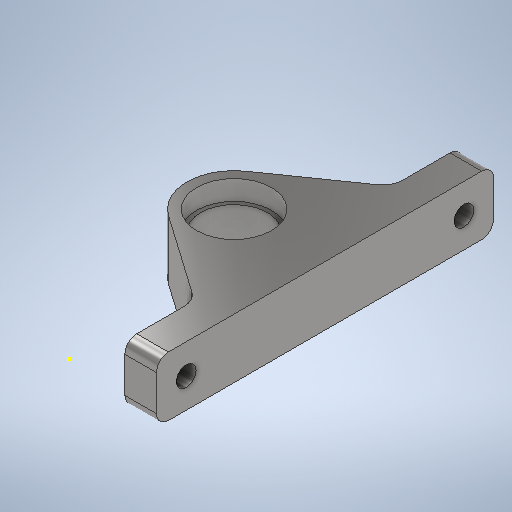
# Autodesk Inventor part: mancal[1]
Saved by Autodesk Inventor 2025 (Build 290162010, 162A)
## iProperties
Created: 2024-09-25
Part Number: mancal[1]
Material: Steel, Mild
Document SubType Name: Modeling
Designer: IFSP
Density: 7.85 g/cm^3
Appearance: Semi-Polished
Author: IFSP
Autodesk Inventor part; units mm, degrees
ref_plane "YZ Plane" through (0, 0, 0) normal (1, 0, 0) x (0, 1, 0)
ref_plane "XZ Plane" through (0, 0, 0) normal (0, 1, 0) x (-1, 0, 0)
ref_plane "XY Plane" through (0, 0, 0) normal (0, 0, 1) x (1, 0, 0)
sketch "Sketch1" plane through (0, 0, 0) normal (0, 1, 0) x (-1, 0, 0)
  circle A0 centre (0, 0) radius 9.45
  circle A1 centre (0, 0) radius 8.45
  line L0 (15.45, 25) -> (15.45, -25)
  line L1 (-20, 0) -> (-15, 0)
  line L2 (-15, 0) -> (-15, 25)
  line L3 (-15, 25) -> (-20, 25)
  line L4 (-20, 25) -> (-20, 0)
  line L5 (-20, 0) -> (-15, 0)
  line L6 (-15, 0) -> (-15, -25)
  line L7 (-15, -25) -> (-20, -25)
  line L8 (-20, -25) -> (-20, 0)
  line L9 (15.45, 25) -> (-20, 25)
  line L10 (-20, 25) -> (-20, -25)
  line L11 (-20, -25) -> (15.45, -25)
  line L12 (15.45, -25) -> (15.45, 25)
  point P0 (15.45, 0)
  dimension "d0" = 18.9
  dimension "d1" = 16.9
  dimension "d7" = 5
  dimension "d8" = 20
  constraints: 26 end point, 6 parallel, 3 horizontal, 3 perpendicular, 2 centre point, 2 coincident
  measures "d0" diameter of A0
  measures "d1" diameter of A1
  measures "d7" distance of L3.end L2.end
  measures "d8" distance from line of L8 point (0, 0)
extrude "Extrusion1" add sketch "Sketch1" along normal blind 10 contours L0 L11 L6 L2 L9 | L2 L1 L4 L3 | L7 L8 L1 L6
extrude "Extrusion2" add sketch "Sketch1" along normal blind 4.9 contours A0
sketch "Sketch2" plane through (0, 10, 0) normal (0, 1, 0) x (1, 0, 0)
  circle A0 centre (0, 0) radius 11.9
  line L0 (-15.45, -25) -> (20, -25) projected
  line L1 (20, 25) -> (-15.45, 25) projected
  line L2 (20, -25) -> (15, -25)
  line L3 (15, -25) -> (15, 25)
  line L4 (15, 25) -> (20, 25)
  line L5 (20, 25) -> (20, -25)
  line L6 (-15.45, 25) -> (-15.45, -25) projected
  line L7 (20, -25) -> (-15.45, -25)
  line L8 (-15.45, -25) -> (-15.45, 25)
  line L9 (-15.45, 25) -> (20, 25)
  line L10 (20, 25) -> (20, -25)
  point P0 (-6.8165, -9.7543)
  point P1 (-6.8165, 9.7543)
  dimension "d13" = 23.8
  dimension "d14" = 5
  constraints: 16 end point, 4 parallel, 2 horizontal, 2 perpendicular, 2 point on circle, 1 centre point, 1 coincident, 1 point on line
  measures "d13" diameter of A0
  measures "d14" distance of L3.end L4.end
sketch "Sketch7" plane through (20, 0, -25) normal (0, 0, -1) x (-1, 0, 0)
  line L0 (35.45, 0) -> (35.45, 10) projected
  line L1 (0, 0) -> (35.45, 0)
  line L2 (35.45, 0) -> (35.45, 10)
  line L3 (35.45, 10) -> (0, 10)
  line L4 (0, 10) -> (0, 0)
  point P0 (20, 0)
  constraints: 8 end point, 2 parallel, 1 horizontal, 1 perpendicular
extrude "Extrusion7" add sketch "Sketch7" along normal blind 10
sketch "Sketch8" plane through (-15.45, 0, 25) normal (0, 0, 1) x (1, 0, 0)
  line L0 (35.45, 0) -> (35.45, 10) projected
  line L1 (0, 0) -> (0, 10) projected
  line L2 (35.45, 0) -> (0, 0)
  line L3 (0, 0) -> (0, 10)
  line L4 (0, 10) -> (35.45, 10)
  line L5 (35.45, 10) -> (35.45, 0)
  point P0 (15.45, 0)
  constraints: 8 end point, 2 parallel, 1 horizontal, 1 perpendicular
extrude "Extrusion8" add sketch "Sketch8" along normal blind 10
sketch "Sketch9" plane through (0, 10, 0) normal (0, 1, 0) x (1, 0, 0)
  circle A0 centre (0, 0) radius 11.9 projected
  line L0 (15, -25) -> (15, 25) projected
  line L1 (15, -25) -> (-6.8165, -9.7543)
  line L2 (15, 25) -> (-6.8165, 9.7543)
  line L3 (20, 35) -> (20, -35) projected
  line L4 (20, 25) -> (15, 25)
  line L5 (15, 25) -> (15, 35)
  line L6 (15, 35) -> (20, 35)
  line L7 (20, 35) -> (20, 25)
  line L8 (20, -25) -> (15, -25)
  line L9 (15, -25) -> (15, -35)
  line L10 (15, -35) -> (20, -35)
  line L11 (20, -35) -> (20, -25)
  line L12 (15, -25) -> (15, 25)
  line L13 (-15.45, -35) -> (-15.45, 35) projected
  line L14 (-15.45, 25) -> (15, 25)
  line L15 (15, -25) -> (-15.45, -25)
  line L16 (-15.45, -25) -> (-15.45, 25)
  line L17 (15, -25) -> (-15.45, -25)
  line L18 (-15.45, -25) -> (-15.45, -35)
  line L19 (-15.45, -35) -> (15, -35)
  line L20 (15, -35) -> (15, -25)
  line L21 (20, 35) -> (-15.45, 35) projected
  line L22 (15, 25) -> (-15.45, 25)
  line L23 (-15.45, 25) -> (-15.45, 35)
  line L24 (-15.45, 35) -> (15, 35)
  line L25 (15, 35) -> (15, 25)
  point P0 (15, 25)
  dimension "d27" = 10
  constraints: 44 end point, 9 parallel, 5 perpendicular, 4 horizontal, 4 point on line, 2 collinear, 2 point on circle, 2 tangent
  measures "d27" distance of L4.end L5.end
extrude "Extrusion9" cut sketch "Sketch9" against normal blind 10 contours A0 L1 L15 L13 L14 L2
extrude "Extrusion10" cut sketch "Sketch9" against normal blind 10 contours L14 L13 L21 L5 | L9 L19 L13 L15
fillet "Fillet1" radius 5 2 edges at (15, 5, 25) (15, 5, -25)
sketch "Sketch10" plane through (-15.45, 0, 35) normal (0, 0, 1) x (1, 0, 0)
  line L0 (35.45, 10) -> (35.45, 0) projected
  line L1 (30.45, 10) -> (30.45, 0) projected
  line L2 (35.45, 0) -> (30.45, 0)
  line L3 (30.45, 0) -> (30.45, 10)
  line L4 (30.45, 10) -> (35.45, 10)
  line L5 (35.45, 10) -> (35.45, 0)
  point P0 (15.45, 0)
  constraints: 8 end point, 2 parallel, 1 horizontal, 1 perpendicular
extrude "Extrusion11" add sketch "Sketch10" along normal blind 2.606
sketch "Sketch11" plane through (20, 0, -35) normal (0, 0, -1) x (-1, 0, 0)
  line L0 (5, 10) -> (0, 10) projected
  line L1 (5, 10) -> (5, 0) projected
  line L2 (0, 10) -> (5, 10)
  line L3 (5, 10) -> (5, 0)
  line L4 (5, 0) -> (0, 0)
  line L5 (0, 0) -> (0, 10)
  point P0 (20, 0)
  constraints: 8 end point, 2 parallel, 1 horizontal, 1 perpendicular
extrude "Extrusion12" add sketch "Sketch11" along normal blind 2.606
sketch "Sketch14" plane through (0, 10, 0) normal (0, 1, 0) x (1, 0, 0)
  circle A0 centre (0, 0) radius 9.45 projected
  line L0 (15, 37.606) -> (15, 27.6058) projected
  arc A1 (12.8641, 23.5074) -> (15, 27.6058) centre (10, 27.6058) ccw projected
  line L1 (12.8641, 23.5074) -> (-6.8165, 9.7543) projected
  arc A2 (-6.8165, 9.7543) -> (-6.8165, -9.7543) centre (0, 0) ccw projected
  line L2 (-6.8165, -9.7543) -> (12.8641, -23.5074) projected
  arc A3 (15, -27.6058) -> (12.8641, -23.5074) centre (10, -27.6058) ccw projected
  line L3 (15, -27.6058) -> (15, -37.606) projected
  line L4 (20, -37.606) -> (15, -37.606) projected
  line L5 (20, 37.606) -> (20, -37.606) projected
  line L6 (15, 37.606) -> (20, 37.606) projected
extrude "Extrusion15" add sketch "Sketch14" along normal blind 2
sketch "Sketch15" plane through (0, 0, 0) normal (0, -1, 0) x (1, 0, 0)
  line L0 (15, -27.6058) -> (15, -37.606) projected
  line L1 (20, -37.606) -> (15, -37.606) projected
  line L2 (20, 37.606) -> (20, -37.606) projected
  line L3 (15, 37.606) -> (20, 37.606) projected
  line L4 (15, 37.606) -> (15, 27.6058) projected
  arc A0 (12.8641, 23.5074) -> (15, 27.6058) centre (10, 27.6058) ccw projected
  line L5 (12.8641, 23.5074) -> (-6.8165, 9.7543) projected
  arc A1 (-6.8165, 9.7543) -> (-6.8165, -9.7543) centre (0, 0) ccw projected
  line L6 (-6.8165, -9.7543) -> (12.8641, -23.5074) projected
  arc A2 (15, -27.6058) -> (12.8641, -23.5074) centre (10, -27.6058) ccw projected
  circle A3 centre (0, 0) radius 8.45 projected
extrude "Extrusion16" add sketch "Sketch15" along normal blind 2
sketch "Sketch16" plane through (0, 4.9, 0) normal (0, 1, 0) x (1, 0, 0)
  circle A0 centre (0, 0) radius 9.45 projected
  circle A1 centre (0, 0) radius 8.45 projected
extrude "Extrusion17" add sketch "Sketch16" along normal blind 2.1
sketch "Sketch17" plane through (-15.45, 0, 37.606) normal (0, 0, 1) x (1, 0, 0)
  line L0 (35.45, 12) -> (35.45, -2) projected
  line L1 (30.45, 12) -> (35.45, 12) projected
  line L2 (30.45, -2) -> (30.45, 12) projected
  line L3 (35.45, -2) -> (30.45, -2) projected
  point P0 (15.45, 0)
extrude "Extrusion18" add sketch "Sketch17" along normal blind 4
sketch "Sketch18" plane through (20, 0, -37.606) normal (0, 0, -1) x (-1, 0, 0)
  line L0 (5, 12) -> (5, -2) projected
  line L1 (0, 12) -> (5, 12) projected
  line L2 (0, -2) -> (0, 12) projected
  line L3 (5, -2) -> (0, -2) projected
  point P0 (20, 0)
extrude "Extrusion19" add sketch "Sketch18" along normal blind 4
sketch "Sketch22" plane through (0, -2, 0) normal (0, -1, 0) x (1, 0, 0)
  arc A0 (-6.8165, 9.7543) -> (-6.8165, -9.7543) centre (0, 0) ccw projected
  line L0 (-6.8165, -9.7543) -> (12.8641, -23.5074) projected
  arc A1 (15, -27.6058) -> (12.8641, -23.5074) centre (10, -27.6058) ccw projected
  line L1 (15, -27.6058) -> (15, -41.606) projected
  line L2 (20, -41.606) -> (15, -41.606) projected
  line L3 (20, 41.606) -> (20, -41.606) projected
  line L4 (15, 41.606) -> (20, 41.606) projected
  line L5 (15, 27.6058) -> (15, 41.606) projected
  arc A2 (12.8641, 23.5074) -> (15, 27.6058) centre (10, 27.6058) ccw projected
  line L6 (12.8641, 23.5074) -> (-6.8165, 9.7543) projected
  circle A3 centre (0, 0) radius 8.45 projected
extrude "Extrusion22" add sketch "Sketch22" along normal blind 1
sketch "Sketch23" plane through (-15.45, 0, 41.606) normal (0, 0, 1) x (1, 0, 0)
  line L0 (30.45, 12) -> (30.45, -3) projected
  line L1 (35.45, -3) -> (30.45, -3) projected
  line L2 (35.45, 12) -> (35.45, -3) projected
  line L3 (35.45, 12) -> (30.45, 12) projected
  line L4 (35.45, 12) -> (35.45, -3) projected
  line L5 (30.45, -3) -> (35.45, -3) projected
  line L6 (30.45, 12) -> (30.45, -3) projected
  line L7 (30.45, 12) -> (35.45, 12) projected
  point P0 (15.45, 0)
sketch "Sketch24" plane through (-15.45, 0, 41.606) normal (0, 0, 1) x (1, 0, 0)
  point P0 (15.45, 0)
extrude "Extrusion23" add sketch "Sketch23" along normal blind 1
sketch "Sketch25" plane through (20, 0, -41.606) normal (0, 0, -1) x (-1, 0, 0)
  line L0 (0, 12) -> (0, -3) projected
  line L1 (5, -3) -> (0, -3) projected
  line L2 (5, 12) -> (5, -3) projected
  line L3 (5, 12) -> (0, 12) projected
  point P0 (20, 0)
extrude "Extrusion24" add sketch "Sketch25" along normal blind 1
sketch "Sketch26" plane through (15, -3, 27.6058) normal (-1, 0, 0) x (0, 0, 1)
  line L0 (0, 0) -> (0, 15) projected
  line L1 (0, 0) -> (15.0002, 0) projected
  line L2 (15.0002, 15) -> (15.0002, 0) projected
  line L3 (0, 15) -> (15.0002, 15) projected
  circle A0 centre (7.5001, 7.5) radius 2.5
  point P0 (-27.6058, 3)
  dimension "d67" = 5
  constraints: 1 centre point
  measures "d67" diameter of A0
extrude "Extrusion25" cut sketch "Sketch26" against normal up to surface (5 mm away) contours A0
sketch "Sketch27" plane through (15, -3, -27.6058) normal (-1, 0, 0) x (0, 0, 1)
  line L0 (0, 15) -> (0, 0) projected
  line L1 (0, 15) -> (-15.0002, 15) projected
  line L2 (-15.0002, 0) -> (-15.0002, 15) projected
  line L3 (0, 0) -> (-15.0002, 0) projected
  circle A0 centre (-7.5001, 7.5) radius 2.5
  point P0 (27.6058, 3)
  dimension "d70" = 5
  constraints: 1 centre point
  measures "d70" diameter of A0
extrude "Extrusion26" cut sketch "Sketch27" against normal up to surface (5 mm away) contours A0
fillet "Fillet4" radius 3 4 edges at (17.5, 12, 42.606) (17.5, -3, 42.606) (17.5, -3, -42.606) (17.5, 12, -42.606)
sketch "Sketch28" plane through (20, 0, 42.606) normal (1, 0, 0) x (0, 0, -1)
  arc A0 (85.212, 9) -> (82.212, 12) centre (82.212, 9) ccw projected
  line L0 (82.212, 12) -> (3, 12) projected
  arc A1 (3, 12) -> (0, 9) centre (3, 9) ccw projected
  line L1 (0, 0) -> (0, 9) projected
  arc A2 (0, 0) -> (3, -3) centre (3, 0) ccw projected
  line L2 (3, -3) -> (82.212, -3) projected
  arc A3 (82.212, -3) -> (85.212, 0) centre (82.212, 0) ccw projected
  line L3 (85.212, 9) -> (85.212, 0) projected
  circle A4 centre (77.7119, 4.5) radius 2.5 projected
  circle A5 centre (7.5001, 4.5) radius 2.5 projected
  point P0 (42.606, 0)
extrude "Extrusion27" add sketch "Sketch28" along normal blind 3
sketch "Sketch29" plane through (0, 12, 0) normal (0, 1, 0) x (1, 0, 0)
  line L0 (15, 39.606) -> (23, 39.606) projected
  line L1 (15, 27.6058) -> (15, 39.606) projected
  arc A0 (12.8641, 23.5074) -> (15, 27.6058) centre (10, 27.6058) ccw projected
  line L2 (12.8641, 23.5074) -> (-6.8165, 9.7543) projected
  arc A1 (-6.8165, 9.7543) -> (-6.8165, -9.7543) centre (0, 0) ccw projected
  line L3 (-6.8165, -9.7543) -> (12.8641, -23.5074) projected
  arc A2 (15, -27.6058) -> (12.8641, -23.5074) centre (10, -27.6058) ccw projected
  line L4 (15, -27.6058) -> (15, -39.606) projected
  line L5 (23, -39.606) -> (15, -39.606) projected
  line L6 (23, 39.606) -> (23, -39.606) projected
  circle A3 centre (0, 0) radius 9.45 projected
  circle A4 centre (0, 0) radius 8.45 projected
  line L7 (15, 39.606) -> (15, 42.606) projected
  line L8 (15, 42.606) -> (23, 42.606) projected
  line L9 (23, 39.606) -> (23, 42.606) projected
  line L10 (15, -42.606) -> (23, -42.606) projected
  line L11 (15, -42.606) -> (15, -39.606) projected
  line L12 (23, -42.606) -> (23, -39.606) projected
  dimension "d76" = 18.9
  dimension "d77" = 16.9
  measures "d76" diameter of A3
  measures "d77" diameter of A4
body "Solid1"
